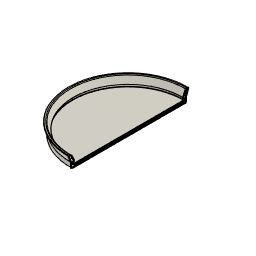
Jogurtové víčko 3 v6 (Autodesk Fusion 360 design; units mm, degrees)
Autodesk Fusion 360 part; units mm, degrees
sketch "Sketch1" plane through (0, 0, 0) normal (0, 1, 0) x (1, 0, 0)
  line L0 (0, 0) -> (-37.75, 0)
  line L1 (-37.75, 0) -> (-40.6618, -8)
  line L2 (-40.6618, -8) -> (-39.0618, -8)
  line L3 (-39.0618, -8) -> (-36.95, -3.5)
  line L4 (-36.95, -3.5) -> (-37.75, -3.5)
  line L5 (-37.75, -3.5) -> (-37.75, -1.6)
  line L6 (-37.75, -1.6) -> (0, -1.6)
  line L7 (0, -1.6) -> (0, 0)
  line L8 (0, -1.6) -> (0, -8)
  line L9 (-39.0239, -3.5) -> (-39.0239, 0)
  line L10 (-39.0239, 0) -> (-37.75, 0)
  dimension "d1" = 75.5
  dimension "d2" = 1.6
  dimension "d3" = 0.8
  dimension "d4" = 1.9
  dimension "d5" = 8
  dimension "d6" = 1.6
  dimension "d7" = 110
  dimension "d9" = 75.5
  constraint coincident L0.start L7.end
  constraint horizontal L0
  constraint parallel L0 L2
  constraint parallel L0 L4
  constraint perpendicular L0 L5
  constraint perpendicular L5 L6
  constraint perpendicular L0 L7
  constraint perpendicular L6 L8
  constraint collinear L7 L8
  constraint coincident L6.end L7.start
  constraint coincident L1 L9.start
  constraint vertical L9
  constraint perpendicular L9 L10
  constraint horizontal L4.end L9.start
  constraint horizontal L2.end L8.end
  measures "d2" distance of L1.end L2.end
  measures "d3" distance of L3.end L4.end
  measures "d4" distance of L4.end L5.end
  measures "d5" distance of L0 L2
  measures "d6" distance of L0 L6
  measures "d7" angle of L0 L1
revolve "Revolve1" add sketch "Sketch1" angle 360 about axis through (0, 0, 1.6) along (0, 0, 1)
chamfer "Chamfer1" distance 0.2 angle 45 1 edges at (-35.1954, 13.651, 1.6)
chamfer "Chamfer2" distance 0.7 distance2 0.4 1 edges at (-35.1954, 13.651, 3.5) measured on face at (11.897, 35.4466, 3.5)
chamfer "Chamfer3" distance 0.4 distance2 0.4 2 edges at (-36.4183, 14.1253, 8) (-37.9101, 14.7039, 8) measured on face at (-39.8316, 3.9607, 8) measured on face at (-39.9165, 3.9942, 6.5)
chamfer "Chamfer4" distance 0.4 distance2 0.4 1 edges at (-36.383, 14.1116, 0) measured on face at (0.5395, 14.867, 0)
equation "d1 = d"
equation "d2 = t"
equation "d3 = x"
equation "d4 = h"
equation "d5 = height"
equation "d6 = t"
equation "d9 = d"
equation "d = 75.5 mm" comment "Průměr víčka"
equation "h = 1.9 mm" comment "Tloušťka víčka"
equation "t = 1.6 mm" comment "Tloušťka stěny"
equation "x = 0.8 mm" comment "Šířka ozubu"
equation "height = 8 mm" comment "Celková výška víčka"
named bodies: "Víčko 3"
